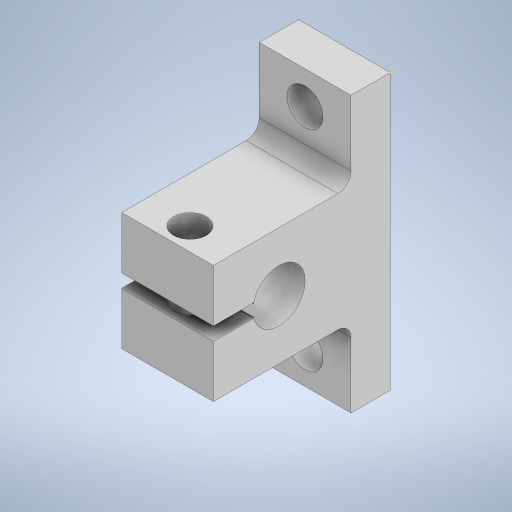
# Autodesk Inventor part: soporte de eje de carril
Saved by Autodesk Inventor 2024.3 (Build 283343000, 343)
## iProperties
Created: 2025-11-05
Part Number: soporte de eje de carril
Material: Generic
Document SubType Name: Modeling
Designer: Windows11
Density: 1 g/cm^3
Appearance: Default
Author: Windows11
Autodesk Inventor part; units mm, degrees
ref_plane "YZ Plane" through (0, 0, 0) normal (1, 0, 0) x (0, 1, 0)
ref_plane "XZ Plane" through (0, 0, 0) normal (0, 1, 0) x (-1, 0, 0)
ref_plane "XY Plane" through (0, 0, 0) normal (0, 0, 1) x (1, 0, 0)
sketch "Sketch1" plane through (0, 0, 0) normal (0, 0, 1) x (1, 0, 0)
  line L0 (0, 0) -> (14, 0)
  line L1 (14, 0) -> (14, -42)
  line L2 (14, -42) -> (0, -42)
  line L3 (0, -42) -> (0, 0)
  dimension "d0" = 14
  dimension "d1" = 42
  constraints: 8 end point, 2 parallel, 1 horizontal, 1 perpendicular
  measures "d0" distance of L1.end L2.end
  measures "d1" distance of L0.end L1.end
extrude "Extrusion1" add sketch "Sketch1" along normal blind 6
sketch "Sketch2" plane through (14, -42, 0) normal (1, 0, 0) x (0, 0, -1)
  line L0 (-6, 30) -> (-27, 30)
  line L1 (-27, 30) -> (-27, 12)
  line L2 (-27, 12) -> (-6, 12)
  line L3 (-6, 12) -> (-6, 30)
  point P0 (0, 42)
  point P1 (-6, 0)
  point P2 (-6, 42)
  constraints: 8 end point, 2 parallel, 1 horizontal, 1 perpendicular
extrude "Extrusion2" add sketch "Sketch2" against normal blind 14
sketch "Sketch3" plane through (14, -42, 0) normal (1, 0, 0) x (0, 0, -1)
  line L0 (0, 42) -> (0, 0) projected
  line L1 (-27, 30) -> (-6, 30) projected
  circle A0 centre (-17, 21) radius 4
  dimension "d11" = 8
  constraints: 1 centre point
  measures "d11" diameter of A0
extrude "Extrusion3" cut sketch "Sketch3" against normal blind 14
sketch "Sketch4" plane through (14, -42, 0) normal (1, 0, 0) x (0, 0, -1)
  point P0 (0, 42)
sketch "Sketch5" plane through (14, -42, 0) normal (1, 0, 0) x (0, 0, -1)
  point P0 (0, 42)
sketch "Sketch6" plane through (0, 0, 0) normal (0, 0, -1) x (-1, 0, 0)
  line L0 (0, -42) -> (-14, -42) projected
  circle A0 centre (-7, -5) radius 2.75
  circle A1 centre (-7, -37) radius 2.75
  point P0 (-14, 0)
  dimension "d16" = 5.5
  dimension "d17" = 5.5
  constraints: 2 centre point
  measures "d16" diameter of A0
  measures "d17" diameter of A1
extrude "Extrusion4" cut sketch "Sketch6" against normal blind 6
sketch "Sketch7" plane through (14, -42, 0) normal (1, 0, 0) x (0, 0, -1)
  point P0 (0, 42)
sketch "Sketch8" plane through (14, -42, 0) normal (1, 0, 0) x (0, 0, -1)
  line L0 (-27, 30) -> (-27, 12) projected
  line L1 (-27, 21) -> (-27, 22)
  line L2 (-27, 21) -> (-27, 20)
  line L3 (-27, 20) -> (-20.908, 20)
  line L4 (-27, 22) -> (-20.908, 22)
  line L5 (-20.908, 22) -> (-20.908, 20)
  point P0 (0, 42)
  dimension "d21" = 1
  constraints: 10 end point, 2 point on line, 1 horizontal, 1 midpoint, 1 perpendicular, 1 vertical
  measures "d21" distance of L1.start L2.end
extrude "Extrusion5" cut sketch "Sketch8" against normal blind 14
sketch "Sketch9" plane through (14, -12, 27) normal (0, 1, 0) x (1, 0, 0)
  line L0 (0, 0) -> (-14, 0) projected
  line L1 (0, 21) -> (-14, 21) projected
  line L2 (-14, 0) -> (-14, 6.092) projected
  circle A0 centre (-7, 3.4183) radius 2.5
  point P0 (-14, 27)
  dimension "d24" = 5
  constraints: 1 centre point
  measures "d24" diameter of A0
extrude "Extrusion6" cut sketch "Sketch9" against normal blind 20
fillet "Fillet1" radius 2 1 edges at (7, -12, 6)
fillet "Fillet2" radius 2 1 edges at (7, -30, 6)
body "Solid1"
